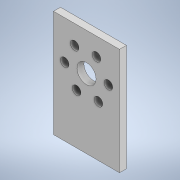
# Autodesk Inventor part: collection motor mount
Saved by Autodesk Inventor 2021 (Build 250183000, 183)
## iProperties
Created: 2021-01-07
Part Number: collection motor mount
Material: Generic
Document SubType Name: Modeling
Designer: User
Density: 1 g/cm^3
Appearance: Default
Author: User
Autodesk Inventor part; units mm, degrees
ref_plane "YZ Plane" through (0, 0, 0) normal (1, 0, 0) x (0, 1, 0)
ref_plane "XZ Plane" through (0, 0, 0) normal (0, 1, 0) x (-1, 0, 0)
ref_plane "XY Plane" through (0, 0, 0) normal (0, 0, 1) x (1, 0, 0)
sketch "Sketch1" plane through (0, 0, 0) normal (0, 0, 1) x (1, 0, 0)
  line L0 (0, 0) -> (24.13, 0)
  line L1 (24.13, 0) -> (24.13, 39.116)
  line L2 (24.13, 39.116) -> (0, 39.116)
  line L3 (0, 39.116) -> (0, 0)
  dimension "d0" = 39.116
  dimension "d1" = 24.13
  constraints: 8 end point, 2 parallel, 1 horizontal, 1 perpendicular
  measures "d0" distance of L0.end L1.end
  measures "d1" distance of L1.end L2.end
extrude "Extrusion1" add sketch "Sketch1" along normal blind 2.54
sketch "Sketch3" plane through (0, 0, 0) normal (0, -1, 0) x (1, 0, 0)
  circle A0 centre (3.9772, 1.2808) radius 0.9652
  circle A1 centre (20.3157, 1.2808) radius 0.9652
  point P0 (0, 0)
  dimension "d7" = 1.9304
  dimension "d8" = 1.9304
  constraints: 2 centre point
  measures "d7" diameter of A0
  measures "d8" diameter of A1
hole "Hole1" at (3.9772, 0, 1.2808) at (20.3157, 0, 1.2808) direction (0, 1, 0) diameter 1.6942 depth 5.7785 tip angle 118 thread size "2-56 UNC" class "2B" standard "ANSI Unified Screw Threads"
sketch "Sketch4" plane through (0, 0, 2.54) normal (0, 0, 1) x (1, 0, 0)
  line L0 (4.7058, 38.0154) -> (12.065, 25.4)
  circle A0 centre (12.065, 25.4) radius 3.4925
  circle A1 centre (12.065, 25.4) radius 8.001
  circle A2 centre (7.7148, 32.1151) radius 1.5875
  circle A3 centre (4.0745, 24.9902) radius 1.5875
  circle A4 centre (12.065, 25.4) radius 8.001
  circle A5 centre (8.4247, 18.2751) radius 1.5875
  circle A6 centre (12.065, 25.4) radius 8.001
  circle A7 centre (16.4152, 18.6849) radius 1.5875
  circle A8 centre (12.065, 25.4) radius 8.001
  circle A9 centre (20.0555, 25.8098) radius 1.5875
  circle A10 centre (12.065, 25.4) radius 8.001
  circle A11 centre (15.7053, 32.5249) radius 1.5875
  circle A12 centre (12.065, 25.4) radius 8.001
  line L1 (24.13, 0) -> (24.13, 39.116) projected
  line L2 (24.13, 39.116) -> (0, 39.116) projected
  line L3 (0, 39.116) -> (0, 0) projected
  line L4 (0, 0) -> (24.13, 0) projected
  dimension "d20" = 16.002
  dimension "d18" = 14.605
  dimension "d19" = 6.985
  dimension "d21" = 3.175
  dimension "d22" = 360
  dimension "d23" = 24.13
  dimension "d24" = 12.065
  dimension "d25" = 25.4
  constraints: 7 centre point, 2 coincident, 2 end point, 43 other
  measures "d18" distance of L0.start L0.end
  measures "d19" diameter of A0
  measures "d21" diameter of A2
  measures "d23" distance of L3.end L1.start
  measures "d24" distance from line of L1 L0.end
  measures "d25" distance from line of A0.centre L4
extrude "Extrusion3" cut sketch "Sketch4" against normal through all contours A2 A1 L0 | L0 A1 A2 | A1 A2 L0 | L0 A2 A1 | A11 A1 | A1 A11 | A3 A1 | A1 A3 | A9 A1 | A1 A9 | A5 A1 | A1 A5 | A7 A1 | A1 A7 | A0
equation "\"d24\" = 0.5 * d23"
body "Solid1"
